makerbeam-10mm-corner v2 (Autodesk Fusion 360 design; units mm, degrees)
Autodesk Fusion 360 part; units mm, degrees
box "BoxPrimitive1" add length 35 width 12 height 12 placed x (0, 0, -1) y (-1, 0, 0) z (0, 1, 0) at (12, 0, 0) makes body 1
box "BoxPrimitive2" add length 12 width 35 height 12 placed x (0, 0, -1) y (-1, 0, 0) z (0, 1, 0) at (35, 0, 0) bodies 1
box "BoxPrimitive3" add length 12 width 12 height 35 placed x (0, 0, -1) y (-1, 0, 0) z (0, 1, 0) at (12, 0, 0) bodies 1
cylinder "CylinderPrimitive1" cut diameter 3 height 15 placed x (1, 0, 0) y (0, 0, -1) z (0, 1, 0) at (30, 0, -5) bodies 1
cylinder "CylinderPrimitive2" cut diameter 3 height 15 placed x (1, 0, 0) y (0, 0, -1) z (0, 1, 0) at (20, 0, -5) bodies 1
cylinder "CylinderPrimitive3" cut diameter 3 height 15 placed x (1, 0, 0) y (0, 0, -1) z (0, 1, 0) at (5, 0, -30) bodies 1
cylinder "CylinderPrimitive4" cut diameter 3 height 15 placed x (1, 0, 0) y (0, 0, -1) z (0, 1, 0) at (5, 0, -20) bodies 1
cylinder "CylinderPrimitive5" cut diameter 3 height 15 placed x (0, 0, -1) y (0, 1, 0) z (1, 0, 0) at (0, 5, -30) bodies 1
cylinder "CylinderPrimitive6" cut diameter 3 height 15 placed x (0, 0, -1) y (0, 1, 0) z (1, 0, 0) at (0, 5, -20) bodies 1
cylinder "CylinderPrimitive7" cut diameter 3 height -15 placed x (0, 1, 0) y (1, 0, 0) z (0, 0, -1) at (30, 5, -12) bodies 1
cylinder "CylinderPrimitive8" cut diameter 3 height -15 placed x (0, 1, 0) y (1, 0, 0) z (0, 0, -1) at (20, 5, -12) bodies 1
cylinder "CylinderPrimitive9" cut diameter 3 height -15 placed x (0, 0, -1) y (0, 1, 0) z (1, 0, 0) at (12, 30, -5) bodies 1
cylinder "CylinderPrimitive10" cut diameter 3 height -15 placed x (0, 0, -1) y (0, 1, 0) z (1, 0, 0) at (12, 20, -5) bodies 1
cylinder "CylinderPrimitive11" cut diameter 3 height -15 placed x (0, 1, 0) y (1, 0, 0) z (0, 0, -1) at (5, 30, -12) bodies 1
cylinder "CylinderPrimitive12" cut diameter 3 height -15 placed x (0, 1, 0) y (1, 0, 0) z (0, 0, -1) at (5, 20, -12) bodies 1
sketch "Sketch24" plane through (0, 0, -12) normal (0, 0, -1) x (-1, 0, 0)
  circle A0 centre (-20, 5) radius 1.5
  circle A1 centre (-30, 5) radius 1.5
  line L0 (-12, 0) -> (-12, 12)
  line L1 (-12, 12) -> (-35, 12)
  line L2 (-35, 12) -> (-35, 0)
  line L3 (-35, 0) -> (-12, 0)
  line L4 (-21.5, 12) -> (-18.5, 12)
  line L5 (-12, 18.5) -> (-12, 21.5)
  line L6 (-20, 12) -> (-12, 20)
  line L7 (-12, 12) -> (-12, 20)
extrude "Extrude5" add sketch "Sketch24" against normal blind 2 separate body contours L1 L4 L5 L6 L7 makes body 2
sketch "Sketch25" plane through (12, 0, 0) normal (1, 0, 0) x (0, 0, -1)
  circle A0 centre (20, 5) radius 1.5
  circle A1 centre (30, 5) radius 1.5
  line L0 (12, 12) -> (12, 0)
  line L1 (12, 0) -> (35, 0)
  line L2 (35, 0) -> (35, 12)
  line L3 (35, 12) -> (12, 12)
  line L4 (12, 20) -> (20, 12)
  line L5 (12, 12) -> (12, 20)
  point P0 (12, 20)
  point P1 (20, 12)
extrude "Extrude6" add sketch "Sketch25" against normal blind 2 separate body contours L3 L4 L5 makes body 3
sketch "Sketch26" plane through (0, 12, 0) normal (0, 1, 0) x (-1, 0, 0)
  circle A0 centre (-5, -20) radius 1.5
  circle A1 centre (-5, -30) radius 1.5
  line L0 (0, -12) -> (-12, -12)
  line L1 (-12, -12) -> (-12, -35)
  line L2 (-12, -35) -> (0, -35)
  line L3 (0, -35) -> (0, -12)
  line L4 (-12, -20) -> (-20, -12)
  line L5 (-20, -12) -> (-12, -12)
  point P0 (-12, -20)
  point P1 (-20, -12)
extrude "Extrude7" add sketch "Sketch26" against normal blind 2 separate body contours L1 L4 L5 makes body 4
box "BoxPrimitive7" cut length 10 width 25 height 10 placed x (0, 0, -1) y (-1, 0, 0) z (0, 1, 0) at (40, 0, 0) bodies 1
box "BoxPrimitive8" cut length 25 width 10 height 10 placed x (0, 0, -1) y (-1, 0, 0) z (0, 1, 0) at (10, 0, -15) bodies 1
box "BoxPrimitive9" cut length 25 width 10 height -10 placed x (0, 1, 0) y (-1, 0, 0) z (0, 0, 1) at (10, 15, 0) bodies 1
